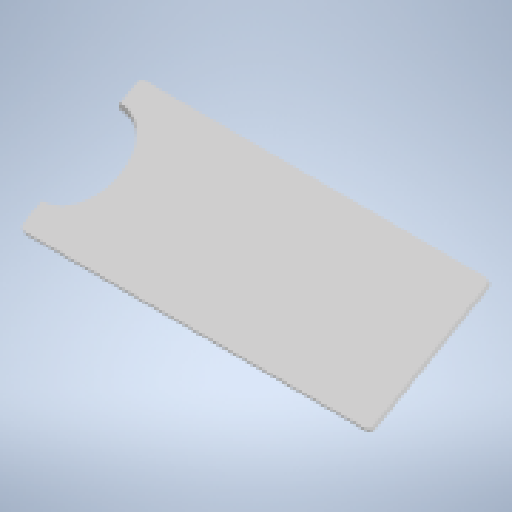
# Autodesk Inventor part: лопасть
Saved by Autodesk Inventor 2023.2 (Build 272271030, 271C)
## iProperties
Created: 2023-08-07
Part Number: лопасть
Material: Stainless Steel
Document SubType Name: Sheet Metal
Designer: admin
Density: 8 g/cm^3
Sheet Metal Rule: Default_mm
Appearance: Default
Flat Pattern Width: 6 cm
Flat Pattern Length: 15 cm
Flat Pattern Area: 90 cm^2
Sheet Metal Width: 60,000 mm
Sheet Metal Length: 150,000 mm
Sheet Metal Area: 9000,000 mm^2
Author: admin
Autodesk Inventor part; units mm, degrees
ref_plane "YZ Plane" through (0, 0, 0) normal (1, 0, 0) x (0, 1, 0)
ref_plane "XZ Plane" through (0, 0, 0) normal (0, 1, 0) x (-1, 0, 0)
ref_plane "XY Plane" through (0, 0, 0) normal (0, 0, 1) x (1, 0, 0)
sketch "Sketch1" plane through (0, 0, 0) normal (1, 0, 0) x (0, 1, 0)
  line L0 (-15.866, 25.4808) -> (14.134, -26.4808)
  line L1 (14.134, -26.4808) -> (15.866, -25.4808)
  line L2 (15.866, -25.4808) -> (-14.134, 26.4808)
  line L3 (-14.134, 26.4808) -> (-15.866, 25.4808)
  line L4 (-15.866, 25.4808) -> (15.866, -25.4808) construction
  line L5 (14.134, -26.4808) -> (-14.134, 26.4808) construction
  line L6 (-15.866, 25.4808) -> (44.134, 25.4808) construction
  point P0 (0, 0)
  dimension "d0" = 60
  dimension "d1" = 60
  dimension "d2" = 2
  constraints: 14 end point, 2 midpoint, 2 parallel, 1 equal length, 1 horizontal, 1 perpendicular
  measures "d0" distance of L0.start L0.end
  measures "d1" angle of L0 L6
  measures "d2" distance of L1.end L0.end
extrude "Extrusion1" add sketch "Sketch1" along normal blind 150
sketch "Sketch2" plane through (0, 0, 0) normal (0, 1, 0) x (-1, 0, 0)
  circle A0 centre (0, 0) radius 16.75
  dimension "d5" = 33.5
  constraints: 1 centre point, 1 coincident
  measures "d5" diameter of A0
extrude "Extrusion2" cut sketch "Sketch2" along normal through all both and the other way through all
fillet "Fillet1" radius 2 4 edges at (150, -15, 25.9808) (150, 15, -25.9808) (0, -15, 25.9808) (0, 15, -25.9808)
equation "\"BendRadius\" = Thickness"
equation "\"BendReliefWidth\" = Thickness"
equation "\"BendReliefDepth\" = 0.5 * Thickness"
equation "\"CornerReliefSize\" = 4 * Thickness"
equation "\"MinimumRemnant\" = 2 * Thickness"
equation "\"TransitionRadius\" = BendRadius"
equation "\"JacobiRadiusSize\" = BendRadius"
equation "\"GapSize\" = Thickness"
equation "\"Thickness\" = 2"
body "Solid1"
